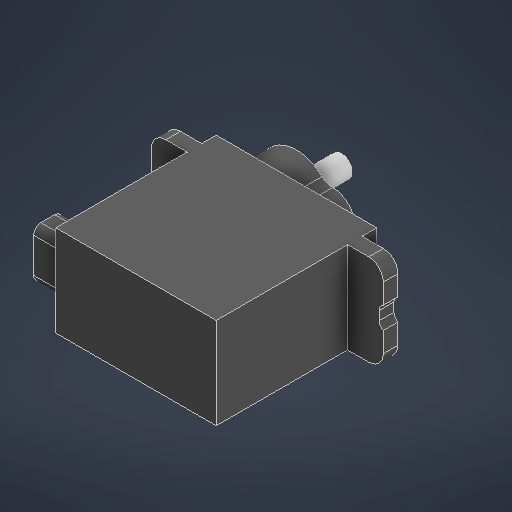
# Autodesk Inventor part: P_Servo_SIMPROP_27x12
Saved by Autodesk Inventor 2026 (Build 300175000, 175)
## iProperties
Created: 2025-08-29
Part Number: P_Servo_SIMPROP_27x12
Material: Generisch
Document SubType Name: Modeling
Designer: FAL
Density: 1.9859 g/cm^3
Appearance: Vorgabe
Mass: 13.6 g
Surface Area: 26.1159 cm^2
Volume: 6.84827 cm^3
Author: FAL
Autodesk Inventor part; units mm, degrees
ref_plane "YZ Plane" through (0, 0, 0) normal (1, 0, 0) x (0, 1, 0)
ref_plane "XZ Plane" through (0, 0, 0) normal (0, 1, 0) x (-1, 0, 0)
ref_plane "XY Plane" through (0, 0, 0) normal (0, 0, 1) x (1, 0, 0)
sketch "Skizze1" plane through (0, 0, 0) normal (0, 1, 0) x (-1, 0, 0)
  line L0 (-11, 6.25) -> (11, 6.25)
  line L1 (11, 6.25) -> (11, -6.25)
  line L2 (11, -6.25) -> (-11, -6.25)
  line L3 (-11, -6.25) -> (-11, 6.25)
  line L4 (-11, 6.25) -> (11, -6.25) construction
  line L5 (11, 6.25) -> (-11, -6.25) construction
  point P0 (0, 0)
  dimension "d0" = 22
  dimension "d1" = 12.5
  constraints: 12 end point, 2 midpoint, 2 parallel, 1 horizontal, 1 perpendicular
  measures "d0" distance of L0.start L0.end
  measures "d1" distance between parallel lines of L2 L0
extrude "Extrusion1" add sketch "Skizze1" along normal blind 22
ref_plane "Arbeitsebene1" through (0, 18, 0) normal (0, 1, 0) x (1, 0, 0)
sketch "Skizze2" plane through (0, 18, 0) normal (0, 1, 0) x (1, 0, 0)
  line L0 (15.9, -6.25) -> (-15.9, -6.25)
  line L1 (-15.9, -6.25) -> (-15.9, 6.25)
  line L2 (-15.9, 6.25) -> (15.9, 6.25)
  line L3 (15.9, 6.25) -> (15.9, -6.25)
  line L4 (15.9, -6.25) -> (-15.9, 6.25) construction
  line L5 (-15.9, -6.25) -> (15.9, 6.25) construction
  line L6 (11, 6.25) -> (-11, 6.25) projected
  point P0 (0, 0)
  dimension "d4" = 31.8
  constraints: 12 end point, 2 midpoint, 2 parallel, 1 collinear, 1 horizontal, 1 perpendicular
  measures "d4" distance between parallel lines of L3 L1
extrude "Extrusion2" add sketch "Skizze2" along normal blind 2
fillet "Rundung1" radius 2 4 edges at (-15.9, 19, 6.25) (15.9, 19, 6.25) (15.9, 19, -6.25) (-15.9, 19, -6.25)
sketch "Skizze3" plane through (0, 22, 0) normal (0, 1, 0) x (1, 0, 0)
  circle A0 centre (-5, 0) radius 5
  circle A1 centre (0, 0) radius 3
  line L0 (-11, 6.25) -> (-11, -6.25) projected
  point P0 (-0.9, -2.8618)
  point P1 (-0.9, 2.8618)
  dimension "d9" = 10
  dimension "d29" = 6
  dimension "d30" = 6
  constraints: 2 horizontal alignment, 1 centre point, 3 other
  measures "d29" diameter of A1
  measures "d30" distance from line of L0 point (-5, 0)
extrude "Extrusion3" add sketch "Skizze3" along normal blind 5
sketch "Skizze5" plane through (0, 22, 0) normal (0, 1, 0) x (1, 0, 0)
  line L0 (15.35, 1.5) -> (16.45, 1.5)
  line L1 (16.45, 1.5) -> (16.45, -1.5)
  line L2 (16.45, -1.5) -> (15.35, -1.5)
  line L3 (15.35, -1.5) -> (15.35, 1.5)
  line L4 (15.9, -4.25) -> (15.9, 4.25) projected
  line L5 (15.35, 1.5) -> (16.45, -1.5) construction
  line L6 (16.45, 1.5) -> (15.35, -1.5) construction
  line L7 (-15.35, 1.5) -> (-16.45, 1.5)
  line L8 (-16.45, 1.5) -> (-16.45, -1.5)
  line L9 (-16.45, -1.5) -> (-15.35, -1.5)
  line L10 (-15.35, -1.5) -> (-15.35, 1.5)
  line L11 (-15.9, 4.25) -> (-15.9, -4.25) projected
  line L12 (-15.35, 1.5) -> (-16.45, -1.5) construction
  line L13 (-16.45, 1.5) -> (-15.35, -1.5) construction
  circle A0 centre (-13.85, 0) radius 1.5 construction
  circle A1 centre (13.85, 0) radius 1.5 construction
  point P0 (0, 0)
  point P1 (15.9, 0)
  point P2 (-15.9, 0)
  dimension "d15" = 3
  dimension "d16" = 3
  dimension "d27" = 27.7
  constraints: 24 end point, 6 midpoint, 6 tangent, 4 parallel, 2 centre point, 2 horizontal, 2 perpendicular, 1 collinear
  measures "d15" distance between parallel lines of L2 L0
  measures "d16" distance between parallel lines of L9 L7
  measures "d27" distance of A0.centre A1.centre
extrude "Extrusion5" cut sketch "Skizze5" against normal blind 5.25
sketch "Skizze4" plane through (-5, 27, 0) normal (0, 1, 0) x (0, 0, 1)
  circle A0 centre (0, 0) radius 1.5
  arc A1 (-2.8618, 4.1) -> (2.8618, 4.1) centre (0, 0) ccw projected
  point P0 (0, 5)
  dimension "d12" = 3
  constraints: 1 centre point, 1 concentric
  measures "d12" diameter of A0
extrude "Extrusion4" add sketch "Skizze4" along normal blind 6.25 separate body
fillet "Rundung2" radius 1 4 edges at (-15.35, 19, -1.5) (-15.35, 19, 1.5) (15.35, 19, 1.5) (15.35, 19, -1.5)
sketch "Skizze6" plane through (-11, 0, -6.25) normal (-1, 0, 0) x (0, 0, 1)
  line L0 (2.1189, 6.0927) -> (8.8811, 6.0927)
  line L1 (8.8811, 6.0927) -> (8.8811, 2.2095)
  line L2 (8.8811, 2.2095) -> (2.1189, 2.2095)
  line L3 (2.1189, 2.2095) -> (2.1189, 6.0927)
  line L4 (2.1189, 6.0927) -> (8.8811, 2.2095) construction
  line L5 (8.8811, 6.0927) -> (2.1189, 2.2095) construction
  point P0 (6.25, 0)
  point P1 (5.5, 4.1511)
  constraints: 12 end point, 2 midpoint, 2 parallel, 1 horizontal, 1 perpendicular
extrude "Extrusion6" add sketch "Skizze6" along normal blind 5.25 bodies 1
fillet "Rundung3" radius 1 4 edges at (-13.625, 6.0927, -4.1311) (-13.625, 2.2095, -4.1311) (-13.625, 2.2095, 2.6311) (-13.625, 6.0927, 2.6311)
fillet "Rundung4" radius 1 8 edges at (-11, 5.7998, 2.3382) (-11, 4.1511, 2.6311) (-11, 2.5023, 2.3382) (-11, 2.2095, -0.75) (-11, 2.5023, -3.8382) (-11, 4.1511, -4.1311) (-11, 5.7998, -3.8382) (-11, 6.0927, -0.75)
fillet "Rundung5" radius 2 2 edges at (-0.9, 24.5, 2.8618) (-0.9, 24.5, -2.8618)
